Autodesk Fusion 360 part; units mm, degrees
note: some values were not read from the file. Set by a fixed rule: which sketch regions a step uses.
(part 4 of 15)
  line L2562 (316.096, -136.511) -> (316.202, -136.249)
  line L2563 (15.562, -135.253) -> (15.8285, -135.16)
  line L2564 (15.8285, -135.16) -> (16.1056, -135.104)
  line L2565 (14.9872, -138.547) -> (14.7954, -138.339)
  line L2566 (316.202, -136.249) -> (316.344, -136.005)
  line L2567 (18.3523, -137.214) -> (18.3147, -137.494)
  line L2568 (318.03, -135.129) -> (318.311, -135.153)
  line L2569 (15.2063, -138.725) -> (14.9872, -138.547)
  line L2570 (316.277, -138.147) -> (316.15, -137.894)
  line L2571 (16.5445, -139.08) -> (16.2621, -139.086)
  line L2572 (18.3147, -137.494) -> (18.238, -137.766)
  line L2573 (14.6348, -138.107) -> (14.5085, -137.854)
  line L2574 (14.877, -135.743) -> (15.0814, -135.548)
  line L2575 (14.5602, -136.209) -> (14.7021, -135.965)
  line L2576 (15.3113, -135.383) -> (15.562, -135.253)
  line L2577 (17.7925, -138.481) -> (17.5821, -138.669)
  line L2578 (17.5821, -138.669) -> (17.3472, -138.826)
  line L2579 (316.01, -137.348) -> (315.999, -137.066)
  line L2580 (17.6789, -135.588) -> (17.8771, -135.79)
  line L2581 (15.9815, -139.053) -> (15.7084, -138.981)
  line L2582 (14.7021, -135.965) -> (14.877, -135.743)
  line L2583 (14.3573, -137.026) -> (14.3861, -136.745)
  line L2584 (18.2769, -136.531) -> (18.3363, -136.807)
  line L2585 (17.2078, -135.279) -> (17.4543, -135.417)
  line L2586 (16.1056, -135.104) -> (16.3877, -135.089)
  line L2587 (18.3363, -136.807) -> (18.3563, -137.089)
  line L2588 (14.4191, -137.586) -> (14.3683, -137.308)
  line L2589 (18.3563, -137.089) -> (18.3523, -137.214)
  line L2590 (316.519, -135.783) -> (316.723, -135.588)
  line L2591 (16.3877, -135.089) -> (16.6691, -135.113)
  line L2592 (14.3861, -136.745) -> (14.4542, -136.471)
  line L2593 (17.3472, -138.826) -> (17.0925, -138.948)
  line L2594 (17.0925, -138.948) -> (16.8232, -139.033)
  line L2595 (16.2621, -139.086) -> (15.9815, -139.053)
  line L2596 (312.976, -138.961) -> (312.791, -138.939)
  line L2597 (313.945, -138.037) -> (313.922, -138.221)
  line L2598 (313.67, -137.341) -> (313.787, -137.485)
  line L2599 (313.772, -138.559) -> (313.651, -138.699)
  line L2600 (312.122, -137.637) -> (312.212, -137.474)
  line L2601 (313.364, -137.135) -> (313.527, -137.223)
  line L2602 (15.7084, -138.981) -> (15.4483, -138.871)
  line L2603 (313.945, -138.011) -> (313.945, -138.037)
  line L2604 (312.791, -138.939) -> (312.615, -138.881)
  line L2605 (14.4542, -136.471) -> (14.5602, -136.209)
  line L2606 (18.1238, -138.025) -> (17.9743, -138.264)
  line L2607 (17.9743, -138.264) -> (17.7925, -138.481)
  line L2608 (313.186, -137.08) -> (313.364, -137.135)
  line L2609 (312.061, -138.182) -> (312.046, -137.998)
  line L2610 (313.863, -138.397) -> (313.772, -138.559)
  line L2611 (312.066, -137.813) -> (312.122, -137.637)
  line L2612 (312.475, -137.216) -> (312.64, -137.13)
  line L2613 (313.922, -138.221) -> (313.863, -138.397)
  line L2614 (312.615, -138.881) -> (312.453, -138.791)
  line L2615 (33.3208, -139.517) -> (33.4627, -139.273)
  line L2616 (37.1129, -140.522) -> (37.0753, -140.802)
  line L2617 (33.3954, -141.415) -> (33.2691, -141.162)
  line L2618 (36.1078, -142.134) -> (35.8531, -142.256)
  line L2619 (36.9986, -141.074) -> (36.8844, -141.333)
  line L2620 (33.556, -141.647) -> (33.3954, -141.415)
  line L2621 (33.1178, -140.334) -> (33.1466, -140.053)
  line L2622 (35.5837, -142.341) -> (35.3051, -142.388)
  line L2623 (33.842, -138.856) -> (34.0719, -138.691)
  line L2624 (293.551, -141.979) -> (293.436, -141.834)
  line L2625 (297.677, -141.687) -> (297.516, -141.455)
  line L2626 (34.0719, -138.691) -> (34.3226, -138.561)
  line L2627 (33.6376, -139.051) -> (33.842, -138.856)
  line L2628 (33.2691, -141.162) -> (33.1797, -140.894)
  line L2629 (297.758, -139.091) -> (297.963, -138.896)
  line L2630 (293.715, -140.524) -> (293.879, -140.438)
  line L2631 (293.3, -141.49) -> (293.285, -141.306)
  line L2632 (293.362, -140.945) -> (293.451, -140.782)
  line L2633 (295.161, -141.529) -> (295.103, -141.705)
  line L2634 (34.2089, -142.179) -> (33.9668, -142.033)
  line L2635 (37.0969, -140.115) -> (37.1169, -140.397)
  line L2636 (297.442, -139.557) -> (297.583, -139.313)
  line L2637 (34.5891, -138.468) -> (34.8662, -138.412)
  line L2638 (35.3051, -142.388) -> (35.0226, -142.394)
  line L2639 (35.8531, -142.256) -> (35.5837, -142.341)
  line L2640 (34.469, -142.289) -> (34.2089, -142.179)
  line L2641 (297.39, -141.202) -> (297.3, -140.934)
  line L2642 (298.443, -138.601) -> (298.71, -138.508)
  line L2643 (36.5531, -141.789) -> (36.3427, -141.977)
  line L2644 (33.1466, -140.053) -> (33.2147, -139.779)
  line L2645 (297.516, -141.455) -> (297.39, -141.202)
  line L2646 (33.1797, -140.894) -> (33.1289, -140.616)
  line L2647 (37.0753, -140.802) -> (36.9986, -141.074)
  line L2648 (33.4627, -139.273) -> (33.6376, -139.051)
  line L2649 (34.7421, -142.361) -> (34.469, -142.289)
  line L2650 (34.3226, -138.561) -> (34.5891, -138.468)
  line L2651 (36.8844, -141.333) -> (36.7349, -141.572)
  line L2652 (299.269, -138.437) -> (299.551, -138.461)
  line L2653 (33.9668, -142.033) -> (33.7478, -141.855)
  line L2654 (33.7478, -141.855) -> (33.556, -141.647)
  line L2655 (36.3427, -141.977) -> (36.1078, -142.134)
  line L2656 (33.2147, -139.779) -> (33.3208, -139.517)
  line L2657 (33.1289, -140.616) -> (33.1178, -140.334)
  line L2658 (36.7349, -141.572) -> (36.5531, -141.789)
  line L2659 (35.0226, -142.394) -> (34.7421, -142.361)
  line L2660 (191.503, -171.203) -> (191.326, -171.146)
  line L2661 (192.238, -169.488) -> (192.381, -169.606)
  line L2662 (192.638, -170.091) -> (192.657, -170.275)
  line L2663 (191.326, -171.146) -> (191.164, -171.056)
  line L2664 (192.585, -169.913) -> (192.638, -170.091)
  line L2665 (322.336, -135.568) -> (322.481, -135.452)
  line L2666 (12.2213, -136.593) -> (12.1297, -136.754)
  line L2667 (322.823, -135.313) -> (323.008, -135.297)
  line L2668 (12.1297, -136.754) -> (12.0086, -136.895)
  line L2669 (322.118, -136.596) -> (322.067, -136.418)
  line L2670 (322.481, -135.452) -> (322.645, -135.366)
  line L2671 (323.008, -135.297) -> (323.192, -135.316)
  line L2672 (12.2798, -136.417) -> (12.2213, -136.593)
  line L2673 (11.8625, -137.009) -> (11.697, -137.092)
  line L2674 (11.697, -137.092) -> (11.5184, -137.142)
  line L2675 (192.05, -171.161) -> (191.872, -171.211)
  line L2676 (11.3336, -137.156) -> (11.1494, -137.134)
  line L2677 (191.898, -169.345) -> (192.075, -169.4)
  line L2678 (192.216, -171.078) -> (192.05, -171.161)
  line L2679 (192.483, -170.823) -> (192.362, -170.963)
  line L2680 (12.3034, -136.207) -> (12.3031, -136.233)
  line L2681 (223.164, -155.286) -> (223.281, -155.43)
  line L2682 (115.359, -156.324) -> (115.589, -156.16)
  line L2683 (115.484, -159.502) -> (115.265, -159.323)
  line L2684 (116.665, -155.866) -> (116.947, -155.89)
  line L2685 (223.021, -155.168) -> (223.164, -155.286)
  line L2686 (222.681, -155.025) -> (222.858, -155.08)
  line L2687 (116.106, -155.936) -> (116.383, -155.881)
  line L2688 (114.912, -158.883) -> (114.786, -158.631)
  line L2689 (114.786, -158.631) -> (114.697, -158.363)
  line L2690 (114.646, -158.085) -> (114.635, -157.803)
  line L2691 (114.98, -156.741) -> (115.155, -156.519)
  line L2692 (223.422, -155.771) -> (223.44, -155.956)
  line L2693 (221.806, -156.616) -> (221.691, -156.47)
  line L2694 (221.691, -156.47) -> (221.606, -156.305)
  line L2695 (221.555, -156.127) -> (221.54, -155.943)
  line L2696 (223.416, -156.166) -> (223.358, -156.342)
  line L2697 (115.155, -156.519) -> (115.359, -156.324)
  line L2698 (114.697, -158.363) -> (114.646, -158.085)
  line L2699 (114.838, -156.985) -> (114.98, -156.741)
  line L2700 (222.858, -155.08) -> (223.021, -155.168)
  line L2701 (223.439, -155.982) -> (223.416, -156.166)
  line L2702 (223.368, -155.594) -> (223.422, -155.771)
  line L2703 (115.589, -156.16) -> (115.84, -156.03)
  line L2704 (116.259, -159.83) -> (115.986, -159.758)
  line L2705 (116.383, -155.881) -> (116.665, -155.866)
  line L2706 (223.281, -155.43) -> (223.368, -155.594)
  line L2707 (222.109, -156.826) -> (221.947, -156.736)
  line L2708 (223.44, -155.956) -> (223.439, -155.982)
  line L2709 (115.265, -159.323) -> (115.073, -159.116)
  line L2710 (223.145, -156.644) -> (222.999, -156.758)
  line L2711 (222.286, -156.884) -> (222.109, -156.826)
  line L2712 (133.779, -149.896) -> (133.938, -150.112)
  line L2713 (221.616, -155.582) -> (221.706, -155.419)
  line L2714 (111.852, -154.785) -> (112.036, -154.768)
  line L2715 (111.157, -155.344) -> (111.246, -155.182)
  line L2716 (112.539, -156.521) -> (112.373, -156.604)
  line L2717 (223.266, -156.503) -> (223.145, -156.644)
  line L2718 (112.821, -155.193) -> (112.908, -155.356)
  line L2719 (112.98, -155.718) -> (112.979, -155.745)
  line L2720 (222.134, -155.075) -> (222.312, -155.023)
  line L2721 (221.947, -156.736) -> (221.806, -156.616)
  line L2722 (222.496, -155.006) -> (222.681, -155.025)
  line L2723 (221.606, -156.305) -> (221.555, -156.127)
  line L2724 (112.221, -154.788) -> (112.398, -154.843)
  line L2725 (112.908, -155.356) -> (112.962, -155.534)
  line L2726 (112.962, -155.534) -> (112.98, -155.718)
  line L2727 (222.312, -155.023) -> (222.496, -155.006)
  line L2728 (221.54, -155.943) -> (221.56, -155.758)
  line L2729 (112.561, -154.931) -> (112.704, -155.049)
  line L2730 (112.979, -155.745) -> (112.956, -155.929)
  line L2731 (222.47, -156.906) -> (222.286, -156.884)
  line L2732 (222.833, -156.841) -> (222.655, -156.891)
  line L2733 (222.655, -156.891) -> (222.47, -156.906)
  line L2734 (221.56, -155.758) -> (221.616, -155.582)
  line L2735 (112.398, -154.843) -> (112.561, -154.931)
  line L2736 (221.969, -155.161) -> (222.134, -155.075)
  line L2737 (112.704, -155.049) -> (112.821, -155.193)
  line L2738 (221.706, -155.419) -> (221.825, -155.277)
  line L2739 (221.825, -155.277) -> (221.969, -155.161)
  line L2740 (222.999, -156.758) -> (222.833, -156.841)
  line L2741 (223.358, -156.342) -> (223.266, -156.503)
  line L2742 (111.08, -155.705) -> (111.101, -155.521)
  line L2743 (111.488, -156.499) -> (111.346, -156.378)
  line L2744 (111.51, -154.924) -> (111.674, -154.838)
  line L2745 (111.346, -156.378) -> (111.231, -156.233)
  line L2746 (111.826, -156.646) -> (111.65, -156.589)
  line L2747 (112.898, -156.105) -> (112.806, -156.266)
  line L2748 (133.377, -149.542) -> (133.59, -149.705)
  line L2749 (133.938, -150.112) -> (134.066, -150.348)
  line L2750 (112.195, -156.654) -> (112.01, -156.668)
  line L2751 (111.095, -155.89) -> (111.08, -155.705)
  line L2752 (112.685, -156.406) -> (112.539, -156.521)
  line L2753 (134.066, -150.348) -> (134.159, -150.6)
  line L2754 (112.806, -156.266) -> (112.685, -156.406)
  line L2755 (112.373, -156.604) -> (112.195, -156.654)
  line L2756 (133.59, -149.705) -> (133.779, -149.896)
  line L2757 (111.231, -156.233) -> (111.147, -156.068)
  line L2758 (111.101, -155.521) -> (111.157, -155.344)
  line L2759 (111.246, -155.182) -> (111.365, -155.04)
  line L2760 (133.143, -149.411) -> (133.377, -149.542)
  line L2761 (111.65, -156.589) -> (111.488, -156.499)
  line L2762 (132.631, -149.253) -> (132.893, -149.314)
  line L2763 (111.674, -154.838) -> (111.852, -154.785)
  line L2764 (112.956, -155.929) -> (112.898, -156.105)
  line L2765 (132.893, -149.314) -> (133.143, -149.411)
  line L2766 (112.01, -156.668) -> (111.826, -156.646)
  line L2767 (111.365, -155.04) -> (111.51, -154.924)
  line L2768 (112.036, -154.768) -> (112.221, -154.788)
  line L2769 (111.147, -156.068) -> (111.095, -155.89)
  line L2770 (203.349, -152.377) -> (203.125, -152.526)
  line L2771 (131.579, -149.386) -> (131.833, -149.297)
  line L2772 (131.833, -149.297) -> (132.096, -149.245)
  line L2773 (132.364, -149.23) -> (132.631, -149.253)
  line L2774 (203.629, -149.642) -> (203.788, -149.858)
  line L2775 (130.763, -150.062) -> (130.929, -149.851)
  line L2776 (203.788, -149.858) -> (203.916, -150.094)
  line L2777 (131.341, -149.51) -> (131.579, -149.386)
  line L2778 (202.481, -148.999) -> (202.743, -149.06)
  line L2779 (130.435, -151.07) -> (130.462, -150.803)
  line L2780 (203.548, -152.198) -> (203.349, -152.377)
  line L2781 (202.743, -149.06) -> (202.993, -149.157)
  line L2782 (134.23, -151.249) -> (134.195, -151.515)
  line L2783 (201.828, -152.742) -> (201.569, -152.674)
  line L2784 (131.471, -152.823) -> (131.241, -152.684)
  line L2785 (130.494, -151.603) -> (130.445, -151.338)
  line L2786 (203.972, -151.52) -> (203.863, -151.765)
  line L2787 (132.778, -152.978) -> (132.513, -153.022)
  line L2788 (204.084, -150.876) -> (204.08, -150.995)
  line L2789 (204.009, -150.346) -> (204.065, -150.608)
  line L2790 (130.628, -150.294) -> (130.763, -150.062)
  line L2791 (130.699, -152.097) -> (130.579, -151.857)
  line L2792 (132.513, -153.022) -> (132.244, -153.028)
  line L2793 (133.033, -152.897) -> (132.778, -152.978)
  line L2794 (133.499, -152.631) -> (133.275, -152.78)
  line L2795 (134.013, -152.019) -> (133.871, -152.247)
  line L2796 (134.159, -150.6) -> (134.215, -150.862)
  line L2797 (131.978, -152.996) -> (131.719, -152.928)
  line L2798 (133.698, -152.452) -> (133.499, -152.631)
  line L2799 (203.44, -149.451) -> (203.629, -149.642)
  line L2800 (133.871, -152.247) -> (133.698, -152.452)
  line L2801 (130.851, -152.318) -> (130.699, -152.097)
  line L2802 (130.527, -150.543) -> (130.628, -150.294)
  line L2803 (132.244, -153.028) -> (131.978, -152.996)
  line L2804 (130.929, -149.851) -> (131.123, -149.666)
  line L2805 (130.579, -151.857) -> (130.494, -151.603)
  line L2806 (130.445, -151.338) -> (130.435, -151.07)
  line L2807 (203.863, -151.765) -> (203.721, -151.993)
  line L2808 (131.241, -152.684) -> (131.033, -152.515)
  line L2809 (202.628, -152.724) -> (202.363, -152.768)
  line L2810 (202.363, -152.768) -> (202.094, -152.774)
  line L2811 (202.993, -149.157) -> (203.227, -149.288)
  line L2812 (131.719, -152.928) -> (131.471, -152.823)
  line L2813 (204.08, -150.995) -> (204.045, -151.261)
  line L2814 (134.234, -151.13) -> (134.23, -151.249)
  line L2815 (133.275, -152.78) -> (133.033, -152.897)
  line L2816 (201.569, -152.674) -> (201.321, -152.569)
  line L2817 (204.045, -151.261) -> (203.972, -151.52)
  line L2818 (134.195, -151.515) -> (134.122, -151.774)
  line L2819 (131.033, -152.515) -> (130.851, -152.318)
  line L2820 (134.215, -150.862) -> (134.234, -151.13)
  line L2821 (134.122, -151.774) -> (134.013, -152.019)
  line L2822 (204.065, -150.608) -> (204.084, -150.876)
  line L2823 (201.321, -152.569) -> (201.091, -152.43)
  line L2824 (131.123, -149.666) -> (131.341, -149.51)
  line L2825 (203.125, -152.526) -> (202.883, -152.643)
  line L2826 (132.096, -149.245) -> (132.364, -149.23)
  line L2827 (203.916, -150.094) -> (204.009, -150.346)
  line L2828 (202.094, -152.774) -> (201.828, -152.742)
  line L2829 (203.721, -151.993) -> (203.548, -152.198)
  line L2830 (202.883, -152.643) -> (202.628, -152.724)
  line L2831 (201.091, -152.43) -> (200.883, -152.261)
  line L2832 (130.462, -150.803) -> (130.527, -150.543)
  line L2833 (201.946, -148.991) -> (202.214, -148.976)
  line L2834 (93.1755, -148.749) -> (93.3096, -148.997)
  line L2835 (200.377, -150.289) -> (200.478, -150.04)
  line L2836 (200.779, -149.597) -> (200.973, -149.412)
  line L2837 (200.701, -152.064) -> (200.549, -151.843)
  line L2838 (200.429, -151.603) -> (200.344, -151.349)
  line L2839 (200.312, -150.549) -> (200.377, -150.289)
  line L2840 (202.214, -148.976) -> (202.481, -148.999)
  line L2841 (200.883, -152.261) -> (200.701, -152.064)
  line L2842 (200.613, -149.808) -> (200.779, -149.597)
  line L2843 (91.7997, -147.845) -> (92.0749, -147.909)
  line L2844 (93.0076, -148.522) -> (93.1755, -148.749)
  line L2845 (203.227, -149.288) -> (203.44, -149.451)
  line L2846 (93.3096, -148.997) -> (93.4074, -149.262)
  line L2847 (200.973, -149.412) -> (201.191, -149.256)
  line L2848 (93.4074, -149.262) -> (93.4669, -149.539)
  line L2849 (200.285, -150.816) -> (200.312, -150.549)
  line L2850 (200.295, -151.084) -> (200.285, -150.816)
  line L2851 (201.191, -149.256) -> (201.429, -149.132)
  line L2852 (201.683, -149.043) -> (201.946, -148.991)
  line L2853 (96.6807, -149.772) -> (96.8578, -149.827)
  line L2854 (91.6751, -151.812) -> (91.3926, -151.818)
  line L2855 (200.344, -151.349) -> (200.295, -151.084)
  line L2856 (90.3368, -151.457) -> (90.1177, -151.278)
  line L2857 (93.4453, -150.226) -> (93.3686, -150.498)
  line L2858 (93.4868, -149.82) -> (93.4829, -149.946)
  line L2859 (90.6925, -147.985) -> (90.9591, -147.891)
  line L2860 (200.478, -150.04) -> (200.613, -149.808)
  line L2861 (92.8095, -148.32) -> (93.0076, -148.522)
  line L2862 (92.3384, -148.011) -> (92.5849, -148.149)
  line L2863 (90.9591, -147.891) -> (91.2362, -147.836)
  line L2864 (92.0749, -147.909) -> (92.3384, -148.011)
  line L2865 (201.429, -149.132) -> (201.683, -149.043)
  line L2866 (93.4829, -149.946) -> (93.4453, -150.226)
  line L2867 (200.549, -151.843) -> (200.429, -151.603)
  line L2868 (92.5849, -148.149) -> (92.8095, -148.32)
  line L2869 (93.4669, -149.539) -> (93.4868, -149.82)
  line L2870 (93.3686, -150.498) -> (93.2544, -150.756)
  line L2871 (89.6391, -150.586) -> (89.5497, -150.318)
  line L2872 (90.0076, -148.474) -> (90.212, -148.279)
  line L2873 (92.2231, -151.68) -> (91.9537, -151.765)
  line L2874 (90.839, -151.713) -> (90.5789, -151.602)
  line L2875 (91.5182, -147.821) -> (91.7997, -147.845)
  line L2876 (93.2544, -150.756) -> (93.1049, -150.996)
  line L2877 (91.2362, -147.836) -> (91.5182, -147.821)
  line L2878 (89.5497, -150.318) -> (89.4989, -150.04)
  line L2879 (89.5847, -149.202) -> (89.6908, -148.941)
  line L2880 (89.6908, -148.941) -> (89.8327, -148.696)
  line L2881 (96.4698, -151.652) -> (96.2857, -151.63)
  line L2882 (96.8578, -149.827) -> (97.0209, -149.915)
  line L2883 (91.3926, -151.818) -> (91.1121, -151.785)
  line L2884 (89.5166, -149.477) -> (89.5847, -149.202)
  line L2885 (95.8063, -151.362) -> (95.6911, -151.217)
  line L2886 (97.4216, -150.518) -> (97.4397, -150.703)
  line L2887 (97.1448, -151.391) -> (96.9987, -151.505)
  line L2888 (92.9231, -151.212) -> (92.7126, -151.401)
  line L2889 (90.4418, -148.115) -> (90.6925, -147.985)
  line L2890 (89.926, -151.071) -> (89.7653, -150.838)
  line L2891 (91.1121, -151.785) -> (90.839, -151.713)
  line L2892 (95.6911, -151.217) -> (95.6064, -151.052)
  line L2893 (96.2857, -151.63) -> (96.1093, -151.573)
  line L2894 (92.7126, -151.401) -> (92.4778, -151.558)
  line L2895 (92.4778, -151.558) -> (92.2231, -151.68)
  line L2896 (90.5789, -151.602) -> (90.3368, -151.457)
  line L2897 (89.4878, -149.758) -> (89.5166, -149.477)
  line L2898 (93.1049, -150.996) -> (92.9231, -151.212)
  line L2899 (89.4989, -150.04) -> (89.4878, -149.758)
  line L2900 (89.8327, -148.696) -> (90.0076, -148.474)
  line L2901 (90.212, -148.279) -> (90.4418, -148.115)
  line L2902 (91.9537, -151.765) -> (91.6751, -151.812)
  line L2903 (90.1177, -151.278) -> (89.926, -151.071)
  line L2904 (89.7653, -150.838) -> (89.6391, -150.586)
  line L2905 (95.6165, -150.328) -> (95.7058, -150.166)
  line L2906 (97.368, -150.341) -> (97.4216, -150.518)
  line L2907 (97.1637, -150.033) -> (97.2809, -150.177)
  line L2908 (96.1338, -149.822) -> (96.3116, -149.769)
  line L2909 (96.3116, -149.769) -> (96.4963, -149.753)
  line L2910 (97.3575, -151.089) -> (97.2659, -151.25)
  line L2911 (96.1093, -151.573) -> (95.9475, -151.483)
  line L2912 (97.4397, -150.703) -> (97.4393, -150.729)
  line L2913 (97.0209, -149.915) -> (97.1637, -150.033)
  line L2914 (97.2659, -151.25) -> (97.1448, -151.391)
  line L2915 (95.9695, -149.908) -> (96.1338, -149.822)
  line L2916 (95.6064, -151.052) -> (95.5553, -150.874)
  line L2917 (95.5397, -150.689) -> (95.5604, -150.505)
  line L2918 (87.434, -148.938) -> (87.4336, -148.965)
  line L2919 (86.649, -149.874) -> (86.4641, -149.888)
  line L2920 (96.4963, -149.753) -> (96.6807, -149.772)
  line L2921 (85.8193, -148.26) -> (85.9638, -148.143)
  line L2922 (95.9475, -151.483) -> (95.8063, -151.362)
  line L2923 (96.9987, -151.505) -> (96.8332, -151.588)
  line L2924 (97.2809, -150.177) -> (97.368, -150.341)
  line L2925 (95.7058, -150.166) -> (95.825, -150.024)
  line L2926 (95.5604, -150.505) -> (95.6165, -150.328)
  line L2927 (87.0152, -148.151) -> (87.1581, -148.269)
  line L2928 (85.9418, -149.718) -> (85.8006, -149.598)
  line L2929 (97.4393, -150.729) -> (97.416, -150.913)
  line L2930 (97.416, -150.913) -> (97.3575, -151.089)
  line L2931 (95.5553, -150.874) -> (95.5397, -150.689)
  line L2932 (87.4336, -148.965) -> (87.4104, -149.149)
  line L2933 (95.825, -150.024) -> (95.9695, -149.908)
  line L2934 (96.8332, -151.588) -> (96.6546, -151.638)
  line L2935 (96.6546, -151.638) -> (96.4698, -151.652)
  line L2936 (87.4104, -149.149) -> (87.3519, -149.325)
  line L2937 (86.8276, -149.824) -> (86.649, -149.874)
  line L2938 (243.907, -149.001) -> (243.697, -149.19)
  line L2939 (243.207, -149.469) -> (242.938, -149.554)
  line L2940 (244.391, -147.051) -> (244.451, -147.327)
  line L2941 (85.8006, -149.598) -> (85.6855, -149.453)
  line L2942 (87.1581, -148.269) -> (87.2753, -148.413)
  line L2943 (243.462, -149.346) -> (243.207, -149.469)
  line L2944 (86.306, -148.005) -> (86.4906, -147.988)
  line L2945 (87.2753, -148.413) -> (87.3623, -148.576)
  line L2946 (242.096, -149.574) -> (241.823, -149.501)
  line L2947 (241.321, -149.246) -> (241.102, -149.067)
  line L2948 (240.91, -148.86) -> (240.749, -148.627)
  line L2949 (241.563, -149.391) -> (241.321, -149.246)
  line L2950 (85.6108, -148.564) -> (85.7002, -148.402)
  line L2951 (244.089, -148.785) -> (243.907, -149.001)
  line L2952 (241.823, -149.501) -> (241.563, -149.391)
  line L2953 (86.28, -149.866) -> (86.1037, -149.809)
  line L2954 (85.5341, -148.925) -> (85.5548, -148.741)
  line L2955 (87.3623, -148.576) -> (87.4159, -148.754)
  line L2956 (87.3519, -149.325) -> (87.2603, -149.486)
  line L2957 (243.793, -146.109) -> (243.992, -146.31)
  line L2958 (243.322, -145.8) -> (243.569, -145.938)
  line L2959 (85.6855, -149.453) -> (85.6007, -149.288)
  line L2960 (240.749, -148.627) -> (240.623, -148.375)
  line L2961 (244.352, -148.287) -> (244.238, -148.545)
  line L2962 (243.697, -149.19) -> (243.462, -149.346)
  line L2963 (85.5548, -148.741) -> (85.6108, -148.564)
  line L2964 (242.784, -145.634) -> (243.059, -145.698)
  line L2965 (86.8522, -148.063) -> (87.0152, -148.151)
  line L2966 (244.238, -148.545) -> (244.089, -148.785)
  line L2967 (86.1037, -149.809) -> (85.9418, -149.718)
  line L2968 (87.4159, -148.754) -> (87.434, -148.938)
  line L2969 (87.2603, -149.486) -> (87.1392, -149.626)
  line L2970 (85.5496, -149.11) -> (85.5341, -148.925)
  line L2971 (242.938, -149.554) -> (242.659, -149.6)
  line L2972 (85.6007, -149.288) -> (85.5496, -149.11)
  line L2973 (243.992, -146.31) -> (244.159, -146.538)
  line L2974 (87.1392, -149.626) -> (86.993, -149.74)
  line L2975 (86.4641, -149.888) -> (86.28, -149.866)
  line L2976 (242.376, -149.607) -> (242.096, -149.574)
  line L2977 (86.675, -148.008) -> (86.8522, -148.063)
  line L2978 (85.9638, -148.143) -> (86.1281, -148.057)
  line L2979 (86.993, -149.74) -> (86.8276, -149.824)
  line L2980 (86.1281, -148.057) -> (86.306, -148.005)
  line L2981 (85.7002, -148.402) -> (85.8193, -148.26)
  line L2982 (244.294, -146.786) -> (244.391, -147.051)
  line L2983 (238.244, -149.039) -> (238.123, -149.179)
  line L2984 (244.451, -147.327) -> (244.471, -147.609)
  line L2985 (238.394, -148.702) -> (238.336, -148.878)
  line L2986 (240.534, -148.107) -> (240.483, -147.829)
  line L2987 (242.22, -145.625) -> (242.502, -145.609)
  line L2988 (237.448, -149.441) -> (237.264, -149.419)
  line L2989 (243.569, -145.938) -> (243.793, -146.109)
  line L2990 (237.977, -149.293) -> (237.811, -149.377)
  line L2991 (241.943, -145.68) -> (242.22, -145.625)
  line L2992 (240.472, -147.546) -> (240.5, -147.265)
  line L2993 (238.142, -147.822) -> (238.259, -147.966)
  line L2994 (240.5, -147.265) -> (240.569, -146.991)
  line L2995 (240.483, -147.829) -> (240.472, -147.546)
  line L2996 (241.426, -145.904) -> (241.676, -145.774)
  line L2997 (237.836, -147.616) -> (237.999, -147.704)
  line L2998 (238.418, -148.518) -> (238.394, -148.702)
  line L2999 (248.148, -146.058) -> (248.265, -146.201)
  line L3000 (238.418, -148.491) -> (238.418, -148.518)
  line L3001 (241.102, -149.067) -> (240.91, -148.86)
  line L3002 (240.623, -148.375) -> (240.534, -148.107)
  line L3003 (238.336, -148.878) -> (238.244, -149.039)
  line L3004 (241.196, -146.068) -> (241.426, -145.904)
  line L3005 (240.817, -146.485) -> (240.991, -146.263)
  line L3006 (244.471, -147.609) -> (244.467, -147.735)
  line L3007 (244.159, -146.538) -> (244.294, -146.786)
  line L3008 (240.991, -146.263) -> (241.196, -146.068)
  line L3009 (243.059, -145.698) -> (243.322, -145.8)
  line L3010 (238.123, -149.179) -> (237.977, -149.293)
  line L3011 (237.264, -149.419) -> (237.088, -149.362)
  line L3012 (240.675, -146.729) -> (240.817, -146.485)
  line L3013 (238.4, -148.307) -> (238.418, -148.491)
  line L3014 (237.633, -149.427) -> (237.448, -149.441)
  line L3015 (244.467, -147.735) -> (244.429, -148.015)
  line L3016 (241.676, -145.774) -> (241.943, -145.68)
  line L3017 (242.502, -145.609) -> (242.784, -145.634)
  line L3018 (240.569, -146.991) -> (240.675, -146.729)
  line L3019 (242.659, -149.6) -> (242.376, -149.607)
  line L3020 (86.4906, -147.988) -> (86.675, -148.008)
  line L3021 (237.811, -149.377) -> (237.633, -149.427)
  line L3022 (237.999, -147.704) -> (238.142, -147.822)
  line L3023 (238.259, -147.966) -> (238.346, -148.129)
  line L3024 (238.346, -148.129) -> (238.4, -148.307)
  line L3025 (237.659, -147.561) -> (237.836, -147.616)
  line L3026 (244.429, -148.015) -> (244.352, -148.287)
  line L3027 (248.005, -145.939) -> (248.148, -146.058)
  line L3028 (192.362, -170.963) -> (192.216, -171.078)
  line L3029 (192.498, -169.75) -> (192.585, -169.913)
  line L3030 (191.164, -171.056) -> (191.023, -170.935)
  line L3031 (192.656, -170.302) -> (192.633, -170.486)
  line L3032 (247.842, -145.851) -> (248.005, -145.939)
  line L3033 (191.687, -171.225) -> (191.503, -171.203)
  line L3034 (247.639, -147.663) -> (247.454, -147.677)
  line L3035 (190.823, -170.625) -> (190.772, -170.447)
  line L3036 (192.075, -169.4) -> (192.238, -169.488)
  line L3037 (247.454, -147.677) -> (247.27, -147.655)
  line L3038 (192.574, -170.662) -> (192.483, -170.823)
  line L3039 (237.475, -147.541) -> (237.659, -147.561)
  line L3040 (248.341, -147.113) -> (248.25, -147.275)
  line L3041 (237.112, -147.611) -> (237.29, -147.558)
  line L3042 (236.785, -149.151) -> (236.669, -149.006)
  line L3043 (248.4, -146.938) -> (248.341, -147.113)
  line L3044 (248.424, -146.727) -> (248.423, -146.754)
  line L3045 (248.265, -146.201) -> (248.352, -146.365)
  line L3046 (248.25, -147.275) -> (248.129, -147.415)
  line L3047 (248.423, -146.754) -> (248.4, -146.938)
  line L3048 (236.803, -147.813) -> (236.948, -147.696)
  line L3049 (236.926, -149.271) -> (236.785, -149.151)
  line L3050 (236.539, -148.294) -> (236.595, -148.117)
  line L3051 (236.595, -148.117) -> (236.684, -147.955)
  line L3052 (248.352, -146.365) -> (248.405, -146.543)
  line L3053 (237.29, -147.558) -> (237.475, -147.541)
  line L3054 (236.533, -148.663) -> (236.518, -148.478)
  line L3055 (247.665, -145.796) -> (247.842, -145.851)
  line L3056 (247.983, -147.529) -> (247.817, -147.613)
  line L3057 (236.948, -147.696) -> (237.112, -147.611)
  line L3058 (236.669, -149.006) -> (236.585, -148.841)
  line L3059 (236.684, -147.955) -> (236.803, -147.813)
  line L3060 (247.817, -147.613) -> (247.639, -147.663)
  line L3061 (191.023, -170.935) -> (190.908, -170.79)
  line L3062 (192.381, -169.606) -> (192.498, -169.75)
  line L3063 (248.405, -146.543) -> (248.424, -146.727)
  line L3064 (236.518, -148.478) -> (236.539, -148.294)
  line L3065 (236.585, -148.841) -> (236.533, -148.663)
  line L3066 (248.129, -147.415) -> (247.983, -147.529)
  line L3067 (237.088, -149.362) -> (236.926, -149.271)
  line L3068 (191.872, -171.211) -> (191.687, -171.225)
  line L3069 (192.657, -170.275) -> (192.656, -170.302)
  line L3070 (192.633, -170.486) -> (192.574, -170.662)
  line L3071 (190.908, -170.79) -> (190.823, -170.625)
  line L3072 (190.772, -170.447) -> (190.757, -170.262)
  line L3073 (208.23, -97.7556) -> (208.251, -97.5713)
  line L3074 (208.976, -98.6967) -> (208.8, -98.6394)
  line L3075 (209.854, -97.0994) -> (209.972, -97.2431)
  line L3076 (208.297, -98.1186) -> (208.246, -97.9403)
  line L3077 (208.8, -98.6394) -> (208.638, -98.5489)
  line L3078 (208.307, -97.3946) -> (208.396, -97.2321)
  line L3079 (210.048, -98.1552) -> (209.957, -98.3165)
  line L3080 (208.396, -97.2321) -> (208.516, -97.0901)
  line L3081 (208.246, -97.9403) -> (208.23, -97.7556)
  line L3082 (208.516, -97.0901) -> (208.66, -96.9739)
  line L3083 (209.689, -98.571) -> (209.524, -98.6546)
  line L3084 (125.339, -98.6643) -> (125.154, -98.6786)
  line L3085 (126.124, -97.7288) -> (126.124, -97.7553)
  line L3086 (125.683, -98.5309) -> (125.518, -98.6145)
  line L3087 (210.13, -97.7688) -> (210.13, -97.7954)
  line L3088 (-7.4754, -95.5282) -> (-7.3124, -95.6164)
  line L3089 (126.124, -97.7553) -> (126.101, -97.9392)
  line L3090 (120.203, -94.8469) -> (120.484, -94.8713)
  line L3091 (-7.1884, -97.0919) -> (-7.3346, -97.2061)
  line L3092 (119.921, -94.8624) -> (120.203, -94.8469)
  line L3093 (126.053, -97.3668) -> (126.106, -97.5443)
  line L3094 (-7.0523, -95.8782) -> (-6.9653, -96.0419)
  line L3095 (209.972, -97.2431) -> (210.059, -97.4068)
  line L3096 (-6.9757, -96.7904) -> (-7.0673, -96.9516)
  line L3097 (124.24, -97.9003) -> (124.224, -97.7155)
  line L3098 (-7.0673, -96.9516) -> (-7.1884, -97.0919)
  line L3099 (125.181, -96.7788) -> (125.365, -96.7982)
  line L3100 (210.059, -97.4068) -> (210.112, -97.5843)
  line L3101 (126.106, -97.5443) -> (126.124, -97.7288)
  line L3102 (124.224, -97.7155) -> (124.245, -97.5313)
  line L3103 (209.524, -98.6546) -> (209.345, -98.7044)
  line L3104 (209.957, -98.3165) -> (209.835, -98.4568)
  line L3105 (125.966, -97.2031) -> (126.053, -97.3668)
  line L3106 (124.632, -98.5089) -> (124.491, -98.3887)
  line L3107 (124.376, -98.2434) -> (124.291, -98.0785)
  line L3108 (209.371, -96.8382) -> (209.548, -96.8931)
  line L3109 (124.291, -98.0785) -> (124.24, -97.9003)
  line L3110 (124.794, -98.5993) -> (124.632, -98.5089)
  line L3111 (209.16, -98.7186) -> (208.976, -98.6967)
  line L3112 (210.112, -97.5843) -> (210.13, -97.7688)
  line L3113 (126.042, -98.1152) -> (125.951, -98.2764)
  line L3114 (126.101, -97.9392) -> (126.042, -98.1152)
  line L3115 (124.301, -97.3545) -> (124.39, -97.1921)
  line L3116 (124.39, -97.1921) -> (124.51, -97.05)
  line L3117 (-7.8635, -97.3537) -> (-8.0476, -97.3318)
  line L3118 (124.654, -96.9339) -> (124.818, -96.848)
  line L3119 (209.002, -96.8357) -> (209.187, -96.8189)
  line L3120 (209.712, -96.9813) -> (209.854, -97.0994)
  line L3121 (208.66, -96.9739) -> (208.824, -96.888)
  line L3122 (210.107, -97.9793) -> (210.048, -98.1552)
  line L3123 (124.51, -97.05) -> (124.654, -96.9339)
  line L3124 (124.97, -98.6566) -> (124.794, -98.5993)
  line L3125 (-8.7269, -96.7537) -> (-8.778, -96.5754)
  line L3126 (-7.1695, -95.7345) -> (-7.0523, -95.8782)
  line L3127 (124.245, -97.5313) -> (124.301, -97.3545)
  line L3128 (208.638, -98.5489) -> (208.497, -98.4288)
  line L3129 (208.251, -97.5713) -> (208.307, -97.3946)
  line L3130 (210.13, -97.7954) -> (210.107, -97.9793)
  line L3131 (208.382, -98.2835) -> (208.297, -98.1186)
  line L3132 (208.497, -98.4288) -> (208.382, -98.2835)
  line L3133 (125.705, -96.9412) -> (125.848, -97.0594)
  line L3134 (125.829, -98.4167) -> (125.683, -98.5309)
  line L3135 (125.518, -98.6145) -> (125.339, -98.6643)
  line L3136 (125.154, -98.6786) -> (124.97, -98.6566)
  line L3137 (125.848, -97.0594) -> (125.966, -97.2031)
  line L3138 (208.824, -96.888) -> (209.002, -96.8357)
  line L3139 (125.542, -96.853) -> (125.705, -96.9412)
  line L3140 (124.491, -98.3887) -> (124.376, -98.2434)
  line L3141 (209.548, -96.8931) -> (209.712, -96.9813)
  line L3142 (125.365, -96.7982) -> (125.542, -96.853)
  line L3143 (125.951, -98.2764) -> (125.829, -98.4167)
  line L3144 (209.345, -98.7044) -> (209.16, -98.7186)
  line L3145 (209.187, -96.8189) -> (209.371, -96.8382)
  line L3146 (209.835, -98.4568) -> (209.689, -98.571)
  line L3147 (-7.3124, -95.6164) -> (-7.1695, -95.7345)
  line L3148 (218.313, -95.6303) -> (218.402, -95.4679)
  line L3149 (218.252, -96.1761) -> (218.236, -95.9913)
  line L3150 (-8.7728, -96.2064) -> (-8.7168, -96.0297)
  line L3151 (-8.6421, -96.9186) -> (-8.7269, -96.7537)
  line L3152 (220.136, -96.0311) -> (220.112, -96.215)
  line L3153 (218.503, -96.6645) -> (218.387, -96.5192)
  line L3154 (124.996, -96.7956) -> (125.181, -96.7788)
  line L3155 (-6.9172, -96.6144) -> (-6.9757, -96.7904)
  line L3156 (219.962, -96.5522) -> (219.841, -96.6925)
  line L3157 (124.818, -96.848) -> (124.996, -96.7956)
  line L3158 (219.351, -96.9401) -> (219.166, -96.9544)
  line L3159 (219.529, -96.8903) -> (219.351, -96.9401)
  line L3160 (-6.8936, -96.404) -> (-6.894, -96.4305)
  line L3161 (-6.9117, -96.2194) -> (-6.8936, -96.404)
  line L3162 (-7.3346, -97.2061) -> (-7.5, -97.2897)
  line L3163 (220.064, -95.6426) -> (220.118, -95.8201)
  line L3164 (-6.9653, -96.0419) -> (-6.9117, -96.2194)
  line L3165 (218.257, -95.8071) -> (218.313, -95.6303)
  line L3166 (-8.778, -96.5754) -> (-8.7935, -96.3907)
  line L3167 (-7.6526, -95.4734) -> (-7.4754, -95.5282)
  line L3168 (220.112, -96.215) -> (220.054, -96.391)
  line L3169 (219.166, -96.9544) -> (218.982, -96.9324)
  line L3170 (220.118, -95.8201) -> (220.136, -96.0046)
  line L3171 (219.841, -96.6925) -> (219.695, -96.8067)
  line L3172 (-7.6786, -97.3395) -> (-7.8635, -97.3537)
  line L3173 (219.86, -95.3352) -> (219.977, -95.4789)
  line L3174 (-8.2239, -97.2745) -> (-8.3858, -97.184)
  line L3175 (-8.1995, -95.5231) -> (-8.0216, -95.4708)
  line L3176 (-8.5083, -95.7252) -> (-8.3638, -95.609)
  line L3177 (-6.894, -96.4305) -> (-6.9172, -96.6144)
  line L3178 (219.717, -95.217) -> (219.86, -95.3352)
  line L3179 (220.136, -96.0046) -> (220.136, -96.0311)
  line L3180 (-8.7168, -96.0297) -> (-8.6274, -95.8672)
  line L3181 (-8.5269, -97.0639) -> (-8.6421, -96.9186)
  line L3182 (-8.0476, -97.3318) -> (-8.2239, -97.2745)
  line L3183 (220.054, -96.391) -> (219.962, -96.5522)
  line L3184 (-8.6274, -95.8672) -> (-8.5083, -95.7252)
  line L3185 (218.387, -96.5192) -> (218.303, -96.3543)
  line L3186 (218.303, -96.3543) -> (218.252, -96.1761)
  line L3187 (-8.7935, -96.3907) -> (-8.7728, -96.2064)
  line L3188 (218.236, -95.9913) -> (218.257, -95.8071)
  line L3189 (-8.3638, -95.609) -> (-8.1995, -95.5231)
  line L3190 (-8.3858, -97.184) -> (-8.5269, -97.0639)
  line L3191 (218.806, -96.8751) -> (218.644, -96.7847)
  line L3192 (-7.837, -95.454) -> (-7.6526, -95.4734)
  line L3193 (-7.5, -97.2897) -> (-7.6786, -97.3395)
  line L3194 (219.977, -95.4789) -> (220.064, -95.6426)
  line L3195 (114.965, -96.8923) -> (114.788, -96.8351)
  line L3196 (114.285, -96.3142) -> (114.234, -96.136)
  line L3197 (115.334, -96.9001) -> (115.149, -96.9143)
  line L3198 (115.824, -96.6525) -> (115.678, -96.7666)
  line L3199 (114.788, -96.8351) -> (114.626, -96.7446)
  line L3200 (219.377, -95.074) -> (219.554, -95.1288)
  line L3201 (114.219, -95.9512) -> (114.239, -95.767)
  line L3202 (115.96, -95.4388) -> (116.047, -95.6025)
  line L3203 (114.234, -96.136) -> (114.219, -95.9512)
  line L3204 (115.537, -95.0887) -> (115.7, -95.1769)
  line L3205 (116.118, -95.991) -> (116.095, -96.175)
  line L3206 (218.666, -95.2096) -> (218.83, -95.1238)
  line L3207 (218.402, -95.4679) -> (218.521, -95.3258)
  line L3208 (-19.9127, -92.9064) -> (-19.7785, -93.1551)
  line L3209 (-20.5033, -92.3065) -> (-20.2787, -92.4779)
  line L3210 (114.813, -95.0837) -> (114.991, -95.0313)
  line L3211 (-20.2787, -92.4779) -> (-20.0805, -92.6792)
  line L3212 (-8.0216, -95.4708) -> (-7.837, -95.454)
  line L3213 (114.239, -95.767) -> (114.295, -95.5903)
  line L3214 (-20.0805, -92.6792) -> (-19.9127, -92.9064)
  line L3215 (218.521, -95.3258) -> (218.666, -95.2096)
  line L3216 (218.83, -95.1238) -> (219.008, -95.0714)
  line L3217 (218.644, -96.7847) -> (218.503, -96.6645)
  line L3218 (-19.6808, -93.4201) -> (-19.6213, -93.6963)
  line L3219 (114.648, -95.1696) -> (114.813, -95.0837)
  line L3220 (-19.7785, -93.1551) -> (-19.6808, -93.4201)
  line L3221 (115.843, -95.2951) -> (115.96, -95.4388)
  line L3222 (-19.8338, -94.9139) -> (-19.9833, -95.1537)
  line L3223 (115.945, -96.5121) -> (115.824, -96.6525)
  line L3224 (116.095, -96.175) -> (116.036, -96.3509)
  line L3225 (116.1, -95.78) -> (116.119, -95.9645)
  line L3226 (114.485, -96.6244) -> (114.37, -96.4791)
  line L3227 (-19.6053, -94.1037) -> (-19.6429, -94.3837)
  line L3228 (114.626, -96.7446) -> (114.485, -96.6244)
  line L3229 (115.7, -95.1769) -> (115.843, -95.2951)
  line L3230 (219.554, -95.1288) -> (219.717, -95.217)
  line L3231 (115.149, -96.9143) -> (114.965, -96.8923)
  line L3232 (116.119, -95.9645) -> (116.118, -95.991)
  line L3233 (114.37, -96.4791) -> (114.285, -96.3142)
  line L3234 (218.982, -96.9324) -> (218.806, -96.8751)
  line L3235 (116.047, -95.6025) -> (116.1, -95.78)
  line L3236 (115.678, -96.7666) -> (115.512, -96.8502)
  line L3237 (219.193, -95.0546) -> (219.377, -95.074)
  line L3238 (116.036, -96.3509) -> (115.945, -96.5121)
  line L3239 (219.695, -96.8067) -> (219.529, -96.8903)
  line L3240 (115.512, -96.8502) -> (115.334, -96.9001)
  line L3241 (115.36, -95.0339) -> (115.537, -95.0887)
  line L3242 (219.008, -95.0714) -> (219.193, -95.0546)
  line L3243 (-15.9434, -95.5482) -> (-16.0895, -95.6623)
  line L3244 (114.504, -95.2858) -> (114.648, -95.1696)
  line L3245 (-23.0806, -92.6321) -> (-22.8762, -92.4371)
  line L3246 (-23.5716, -93.6342) -> (-23.5035, -93.3601)
  line L3247 (-21.9761, -95.9427) -> (-22.2492, -95.8703)
  line L3248 (-21.0133, -92.0665) -> (-20.7498, -92.1684)
  line L3249 (-22.6463, -92.2728) -> (-22.3956, -92.1426)
  line L3250 (-17.4818, -95.2099) -> (-17.5329, -95.0317)
  line L3251 (-21.1345, -95.9228) -> (-21.4131, -95.9692)
  line L3252 (-17.5329, -95.0317) -> (-17.5484, -94.847)
  line L3253 (-25.7258, -92.7339) -> (-25.6723, -92.9114)
  line L3254 (-26.0729, -92.3084) -> (-25.9301, -92.4266)
  line L3255 (-17.2632, -94.1815) -> (-17.1187, -94.0653)
  line L3256 (-20.6104, -95.7153) -> (-20.8651, -95.8376)
  line L3257 (-17.2819, -95.5201) -> (-17.3971, -95.3748)
  line L3258 (114.385, -95.4278) -> (114.504, -95.2858)
  line L3259 (-20.7498, -92.1684) -> (-20.5033, -92.3065)
  line L3260 (-17.1407, -95.6403) -> (-17.2819, -95.5201)
  line L3261 (-15.6721, -95.0707) -> (-15.7307, -95.2466)
  line L3262 (-22.5093, -95.7601) -> (-22.7514, -95.6144)
  line L3263 (-19.6013, -93.9781) -> (-19.6053, -94.1037)
  line L3264 (-19.6429, -94.3837) -> (-19.7196, -94.6556)
  line L3265 (-22.7514, -95.6144) -> (-22.9704, -95.436)
  line L3266 (-16.0895, -95.6623) -> (-16.255, -95.7459)
  line L3267 (114.295, -95.5903) -> (114.385, -95.4278)
  line L3268 (-21.852, -91.9939) -> (-21.5699, -91.9783)
  line L3269 (-19.6213, -93.6963) -> (-19.6013, -93.9781)
  line L3270 (-15.6485, -94.8602) -> (-15.6489, -94.8867)
  line L3271 (-21.2885, -92.0027) -> (-21.0133, -92.0665)
  line L3272 (114.991, -95.0313) -> (115.175, -95.0145)
  line L3273 (-22.2492, -95.8703) -> (-22.5093, -95.7601)
  line L3274 (-23.5893, -94.1976) -> (-23.6004, -93.9153)
  line L3275 (-22.3956, -92.1426) -> (-22.1291, -92.049)
  line L3276 (-23.5385, -94.4755) -> (-23.5893, -94.1976)
  line L3277 (-16.2304, -93.9844) -> (-16.0673, -94.0726)
  line L3278 (-23.2555, -92.8539) -> (-23.0806, -92.6321)
  line L3279 (-17.5278, -94.6627) -> (-17.4717, -94.486)
  line L3280 (-21.4131, -95.9692) -> (-21.6956, -95.9759)
  line L3281 (-23.3974, -93.0982) -> (-23.2555, -92.8539)
  line L3282 (-21.6956, -95.9759) -> (-21.9761, -95.9427)
  line L3283 (-20.8651, -95.8376) -> (-21.1345, -95.9228)
  line L3284 (-22.9704, -95.436) -> (-23.1622, -95.2286)
  line L3285 (-15.7307, -95.2466) -> (-15.8222, -95.4078)
  line L3286 (-20.3755, -95.5584) -> (-20.6104, -95.7153)
  line L3287 (-23.1622, -95.2286) -> (-23.3228, -94.9962)
  line L3288 (-16.0673, -94.0726) -> (-15.9244, -94.1908)
  line L3289 (-15.8072, -94.3345) -> (-15.7202, -94.4982)
  line L3290 (-20.1651, -95.3699) -> (-20.3755, -95.5584)
  line L3291 (-21.5699, -91.9783) -> (-21.2885, -92.0027)
  line L3292 (-15.6666, -94.6757) -> (-15.6485, -94.8602)
  line L3293 (-19.7196, -94.6556) -> (-19.8338, -94.9139)
  line L3294 (-15.9244, -94.1908) -> (-15.8072, -94.3345)
  line L3295 (115.175, -95.0145) -> (115.36, -95.0339)
  line L3296 (-15.6489, -94.8867) -> (-15.6721, -95.0707)
  line L3297 (-23.6004, -93.9153) -> (-23.5716, -93.6342)
  line L3298 (-15.7202, -94.4982) -> (-15.6666, -94.6757)
  line L3299 (-15.8222, -95.4078) -> (-15.9434, -95.5482)
  line L3300 (-23.3228, -94.9962) -> (-23.4491, -94.7435)
  line L3301 (-22.8762, -92.4371) -> (-22.6463, -92.2728)
  line L3302 (-22.1291, -92.049) -> (-21.852, -91.9939)
  line L3303 (-19.9833, -95.1537) -> (-20.1651, -95.3699)
  line L3304 (-23.4491, -94.7435) -> (-23.5385, -94.4755)
  line L3305 (-23.5035, -93.3601) -> (-23.3974, -93.0982)
  line L3306 (-16.4075, -93.9296) -> (-16.2304, -93.9844)
  line L3307 (121.608, -98.2385) -> (121.397, -98.427)
  line L3308 (119.263, -98.6287) -> (119.021, -98.4829)
  line L3309 (121.939, -97.7825) -> (121.789, -98.0222)
  line L3310 (118.692, -95.5006) -> (118.897, -95.3056)
  line L3311 (120.36, -98.8378) -> (120.077, -98.8444)
  line L3312 (122.13, -97.2522) -> (122.053, -97.5241)
  line L3313 (120.638, -98.7914) -> (120.36, -98.8378)
  line L3314 (119.021, -98.4829) -> (118.802, -98.3046)
  line L3315 (120.077, -98.8444) -> (119.797, -98.8112)
  line L3316 (118.324, -97.612) -> (118.234, -97.344)
  line L3317 (121.397, -98.427) -> (121.162, -98.5839)
  line L3318 (118.183, -97.0661) -> (118.172, -96.7838)
  line L3319 (118.802, -98.3046) -> (118.611, -98.0971)
  line L3320 (118.234, -97.344) -> (118.183, -97.0661)
  line L3321 (120.908, -98.7062) -> (120.638, -98.7914)
  line L3322 (118.611, -98.0971) -> (118.45, -97.8647)
  line L3323 (121.162, -98.5839) -> (120.908, -98.7062)
  line L3324 (118.201, -96.5028) -> (118.269, -96.2286)
  line L3325 (119.644, -94.9175) -> (119.921, -94.8624)
  line L3326 (118.897, -95.3056) -> (119.126, -95.1414)
  line L3327 (122.167, -96.9722) -> (122.13, -97.2522)
  line L3328 (119.797, -98.8112) -> (119.524, -98.7388)
  line L3329 (118.172, -96.7838) -> (118.201, -96.5028)
  line L3330 (38.3306, -123.634) -> (38.0501, -123.601)
  line L3331 (36.4258, -121.573) -> (36.4546, -121.292)
  line L3332 (37.2748, -123.272) -> (37.0558, -123.094)
  line L3333 (38.6131, -123.627) -> (38.3306, -123.634)
  line L3334 (291.118, -121.628) -> (291.295, -121.683)
  line L3335 (291.703, -123.106) -> (291.582, -123.246)
  line L3336 (291.436, -123.36) -> (291.27, -123.444)
  line L3337 (36.4877, -122.133) -> (36.4369, -121.856)
  line L3338 (290.546, -123.429) -> (290.385, -123.338)
  line L3339 (291.795, -122.945) -> (291.703, -123.106)
  line L3340 (291.859, -122.374) -> (291.877, -122.558)
  line L3341 (37.6306, -119.801) -> (37.8971, -119.707)
  line L3342 (291.295, -121.683) -> (291.458, -121.771)
  line L3343 (291.601, -121.889) -> (291.718, -122.033)
  line L3344 (37.3799, -119.931) -> (37.6306, -119.801)
  line L3345 (40.3066, -122.314) -> (40.1924, -122.572)
  line L3346 (291.876, -122.585) -> (291.853, -122.769)
  line L3347 (290.243, -123.218) -> (290.128, -123.073)
  line L3348 (291.805, -122.196) -> (291.859, -122.374)
  line L3349 (290.907, -123.508) -> (290.723, -123.486)
  line L3350 (38.1742, -119.652) -> (38.4563, -119.636)
  line L3351 (38.0501, -123.601) -> (37.777, -123.528)
  line L3352 (36.5771, -122.401) -> (36.4877, -122.133)
  line L3353 (40.3833, -122.042) -> (40.3066, -122.314)
  line L3354 (40.0429, -122.812) -> (39.8611, -123.028)
  line L3355 (291.718, -122.033) -> (291.805, -122.196)
  line L3356 (290.128, -123.073) -> (290.044, -122.908)
  line L3357 (261.846, -123.067) -> (261.731, -122.922)
  line L3358 (290.054, -122.184) -> (290.143, -122.022)
  line L3359 (44.3541, -122.729) -> (44.2955, -122.905)
  line L3360 (262.897, -121.531) -> (263.06, -121.62)
  line L3361 (263.479, -122.434) -> (263.456, -122.618)
  line L3362 (262.509, -123.357) -> (262.325, -123.335)
  line L3363 (263.407, -122.045) -> (263.461, -122.223)
  line L3364 (42.8855, -123.298) -> (42.7443, -123.178)
  line L3365 (263.397, -122.794) -> (263.305, -122.955)
  line L3366 (262.694, -123.343) -> (262.509, -123.357)
  line L3367 (42.6291, -123.033) -> (42.5444, -122.868)
  line L3368 (262.72, -121.477) -> (262.897, -121.531)
  line L3369 (44.204, -123.066) -> (44.0828, -123.206)
  line L3370 (44.3777, -122.518) -> (44.3773, -122.545)
  line L3371 (42.5444, -122.868) -> (42.4933, -122.69)
  line L3372 (290.571, -121.677) -> (290.749, -121.625)
  line L3373 (44.2955, -122.905) -> (44.204, -123.066)
  line L3374 (43.9367, -123.32) -> (43.7712, -123.404)
  line L3375 (290.262, -121.88) -> (290.407, -121.763)
  line L3376 (290.385, -123.338) -> (290.243, -123.218)
  line L3377 (291.458, -121.771) -> (291.601, -121.889)
  line L3378 (291.877, -122.558) -> (291.876, -122.585)
  line L3379 (290.044, -122.908) -> (289.992, -122.73)
  line L3380 (38.4563, -119.636) -> (38.7377, -119.661)
  line L3381 (36.9456, -120.29) -> (37.15, -120.095)
  line L3382 (291.27, -123.444) -> (291.092, -123.494)
  line L3383 (291.853, -122.769) -> (291.795, -122.945)
  line L3384 (290.723, -123.486) -> (290.546, -123.429)
  line L3385 (43.4078, -123.468) -> (43.2237, -123.446)
  line L3386 (44.3773, -122.545) -> (44.3541, -122.729)
  line L3387 (43.6187, -121.588) -> (43.7958, -121.642)
  line L3388 (43.2237, -123.446) -> (43.0473, -123.389)
  line L3389 (43.7712, -123.404) -> (43.5926, -123.454)
  line L3390 (43.0473, -123.389) -> (42.8855, -123.298)
  line L3391 (42.4778, -122.505) -> (42.4984, -122.321)
  line L3392 (43.2497, -121.585) -> (43.4343, -121.568)
  line L3393 (44.1018, -121.849) -> (44.219, -121.993)
  line L3394 (43.7958, -121.642) -> (43.9589, -121.731)
  line L3395 (37.15, -120.095) -> (37.3799, -119.931)
  line L3396 (290.407, -121.763) -> (290.571, -121.677)
  line L3397 (263.461, -122.223) -> (263.479, -122.407)
  line L3398 (44.306, -122.156) -> (44.3596, -122.334)
  line L3399 (263.456, -122.618) -> (263.397, -122.794)
  line L3400 (261.646, -122.757) -> (261.595, -122.579)
  line L3401 (289.977, -122.545) -> (289.998, -122.361)
  line L3402 (289.998, -122.361) -> (290.054, -122.184)
  line L3403 (290.749, -121.625) -> (290.933, -121.608)
  line L3404 (42.4933, -122.69) -> (42.4778, -122.505)
  line L3405 (290.933, -121.608) -> (291.118, -121.628)
  line L3406 (289.992, -122.73) -> (289.977, -122.545)
  line L3407 (42.763, -121.839) -> (42.9075, -121.723)
  line L3408 (291.092, -123.494) -> (290.907, -123.508)
  line L3409 (37.8971, -119.707) -> (38.1742, -119.652)
  line L3410 (44.3596, -122.334) -> (44.3777, -122.518)
  line L3411 (42.7443, -123.178) -> (42.6291, -123.033)
  line L3412 (291.582, -123.246) -> (291.436, -123.36)
  line L3413 (44.0828, -123.206) -> (43.9367, -123.32)
  line L3414 (262.325, -123.335) -> (262.149, -123.278)
  line L3415 (43.9589, -121.731) -> (44.1018, -121.849)
  line L3416 (261.731, -122.922) -> (261.646, -122.757)
  line L3417 (290.143, -122.022) -> (290.262, -121.88)
  line L3418 (43.4343, -121.568) -> (43.6187, -121.588)
  line L3419 (44.219, -121.993) -> (44.306, -122.156)
  line L3420 (43.5926, -123.454) -> (43.4078, -123.468)
  line L3421 (71.6213, -123.295) -> (71.445, -123.238)
  line L3422 (72.7753, -122.367) -> (72.775, -122.394)
  line L3423 (72.6166, -121.841) -> (72.7037, -122.005)
  line L3424 (261.987, -123.187) -> (261.846, -123.067)
  line L3425 (263.203, -121.738) -> (263.32, -121.881)
  line L3426 (263.038, -123.209) -> (262.873, -123.293)
  line L3427 (71.142, -123.027) -> (71.0268, -122.882)
  line L3428 (72.7037, -122.005) -> (72.7572, -122.183)
  line L3429 (262.173, -121.526) -> (262.351, -121.474)
  line L3430 (42.6438, -121.982) -> (42.763, -121.839)
  line L3431 (261.864, -121.728) -> (262.009, -121.612)
  line L3432 (261.656, -122.033) -> (261.745, -121.87)
  line L3433 (72.3344, -123.169) -> (72.1689, -123.253)
  line L3434 (282.565, -120.988) -> (282.619, -121.166)
  line L3435 (262.536, -121.457) -> (262.72, -121.477)
  line L3436 (71.445, -123.238) -> (71.2832, -123.147)
  line L3437 (282.463, -121.898) -> (282.342, -122.038)
  line L3438 (263.184, -123.095) -> (263.038, -123.209)
  line L3439 (282.619, -121.166) -> (282.637, -121.35)
  line L3440 (281.878, -120.42) -> (282.055, -120.475)
  line L3441 (70.8961, -122.17) -> (70.9522, -121.993)
  line L3442 (71.6473, -121.434) -> (71.832, -121.417)
  line L3443 (282.055, -120.475) -> (282.218, -120.563)
  line L3444 (72.6932, -122.754) -> (72.6016, -122.915)
  line L3445 (71.2832, -123.147) -> (71.142, -123.027)
  line L3446 (72.7517, -122.578) -> (72.6932, -122.754)
  line L3447 (282.03, -122.236) -> (281.852, -122.286)
  line L3448 (281.852, -122.286) -> (281.667, -122.3)
  line L3449 (261.595, -122.579) -> (261.579, -122.394)
  line L3450 (71.4695, -121.486) -> (71.6473, -121.434)
  line L3451 (263.305, -122.955) -> (263.184, -123.095)
  line L3452 (71.9903, -123.303) -> (71.8054, -123.317)
  line L3453 (72.6016, -122.915) -> (72.4805, -123.055)
  line L3454 (72.1935, -121.491) -> (72.3566, -121.58)